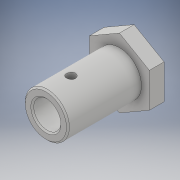
# Autodesk Inventor part: И7-22
Saved by Autodesk Inventor 2019.3 (Build 233278000, 278)
## iProperties
Created: 2020-03-25
Part Number: И7-22
Material: Типовые
Document SubType Name: Modeling
Designer: Admin
Density: 1 g/cm^3
Appearance: По умолчанию
Author: Admin
Autodesk Inventor part; units mm, degrees
ref_plane "YZ Plane" through (0, 0, 0) normal (1, 0, 0) x (0, 1, 0)
ref_plane "XZ Plane" through (0, 0, 0) normal (0, 1, 0) x (-1, 0, 0)
ref_plane "XY Plane" through (0, 0, 0) normal (0, 0, 1) x (1, 0, 0)
sketch "Эскиз1" plane through (0, 0, 0) normal (0, 0, 1) x (1, 0, 0)
  line L0 (0, 23.5) -> (20.3516, 11.75)
  line L1 (20.3516, 11.75) -> (20.3516, -11.75)
  line L2 (20.3516, -11.75) -> (0, -23.5)
  line L3 (0, -23.5) -> (-20.3516, -11.75)
  line L4 (-20.3516, -11.75) -> (-20.3516, 11.75)
  line L5 (-20.3516, 11.75) -> (0, 23.5)
  point P0 (0, 0)
  point P1 (0, 0)
  dimension "d0" = 47
  constraints: 12 end point, 1 coincident, 1 vertical alignment, 13 other
  measures "d0" distance of L2.end L0.start
extrude "Выдавливание1" add sketch "Эскиз1" along normal blind 10
sketch "Эскиз2" plane through (0, 0, 10) normal (0, 0, 1) x (1, 0, 0)
  circle A0 centre (0, 0) radius 15
  dimension "d3" = 30
  constraints: 1 centre point, 1 coincident
  measures "d3" diameter of A0
extrude "Выдавливание2" add sketch "Эскиз2" along normal blind 50
sketch "Эскиз3" plane through (0, 0, 60) normal (0, 0, 1) x (1, 0, 0)
  point P0 (0, 0)
  point P1 (0, 0)
  constraints: 1 coincident
hole "Отверстие1" at (0, 0, 60) direction (0, 0, -1) diameter 18.5 depth 30 tip angle 120
sketch "Эскиз4" plane through (0, 0, 0) normal (0, 0, -1) x (-1, 0, 0)
  point P0 (0, 0)
  point P1 (0, 0)
  constraints: 1 coincident
hole "Отверстие2" at (0, 0, 0) direction (0, 0, 1) diameter 10 end through all
sketch "Эскиз5" plane through (0, 0, 0) normal (0, 1, 0) x (-1, 0, 0)
  circle A0 centre (0, 43) radius 3
  line L0 (15, 60) -> (-15, 60) projected
  point P0 (0, 0)
  dimension "d20" = 6
  dimension "d21" = 17
  constraints: 1 centre point, 1 vertical alignment
  measures "d20" diameter of A0
  measures "d21" distance from line of L0 A0.centre
extrude "Выдавливание3" cut sketch "Эскиз5" along normal through all both and the other way through all
chamfer "Фаска1" distance 1 angle 45 3 edges at (0, 9.25, 60) (-15, 0, 60) (0, -5, 0)
